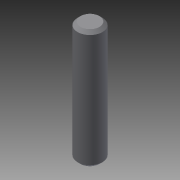
# Autodesk Inventor part: FO-020.751.194NT-00_rod-bif
Saved by Autodesk Inventor 2014 SP2 (Build 180246200, 246)
## iProperties
Created: 2020-02-04
Part Number: FO-020.751.194NT-00_rod-bif
Material: Generic
Catalog Web Link: www.cadenas.de
Description: FO1 Basic Model Rod-Bimba FLAT-1
Vendor: BIMBA
Document SubType Name: Modeling
Designer: psadmin
Manufacturer: BIMBA
Mass: 0.949795 g
Surface Area: 6.49027 cm^2
Volume: 0.949795 cm^3
Density: 1 g/cm^3
Appearance: PSOLRGB-180-180-180
Category: PARTsolutions
Company: BIMBA
Title: FO-020.751.194NT-00_rod-bif
Author: Cadenas PARTsolutions
Comments: Bimba FLAT-1
PSOL_IDENT_0: {$CADENAS_DATA\23d-libs\bimba\bimba_brand\bimba_imperial\bimba_full_line\flat_cylinders\fo1\fo1_basi
PSOL_IDENT_1: c_model_rod.prj},304 {VTYP=3D},{NB=FO-020.751.194NT-00_rod-bif},{LINA=FO-020.751.194NT-00_rod-bif},{
PSOL_IDENT_2: NN=FO1 Basic Model Rod},{DATE=22.01.2020 09:06:03},{GEOMDATE=12.12.2018 07:59:21},{VERSION=},{LINEID=
PSOL_IDENT_3: 10},{WBVAR=STROKE,ACTING,MNTR,MNTF,HR,FS,LENGTH,STPT1,STPT2,STPT3,RT,M,W,UM,MRS,FCD,RCD},{WBNUMERIC=
PSOL_IDENT_4: STROKE,LENGTH,FCD,RCD}  {NB=FO-020.751.194NT-00_rod-bif},{LINA=FO-020.751.194NT-00_rod-bif},{KT=DUMM
PSOL_IDENT_5: Y},{PN=FO-020.751.194NT-00},{PN2=FO-020.751.194NT-00},{BORE=0.56250000},{BOREPN=02},{BORE1=0.562},{S
PSOL_IDENT_6: TROKE=0.75000},{STROKEMIN=0.61},{STROKEMAX=16},{ACTING=},{ACTINGALG='','Double Acting, Single End Ro
PSOL_IDENT_7: d [FO]', 'D'  , 'Double Acting, Double End Rod [FOD]', 'R', 'Reverse Acting [FOR]', 'S'  ,'Single Ac
PSOL_IDENT_8: ting [FOS]'},{MNTR=},{MNTF=},{MNTFALG='','Standard Counterbored Mounting Holes','2F','Trunnion Mount
PSOL_IDENT_9: , Front','3F','Threaded Mounting Holes, Front','4F','Screw Clearance Holes, Front','5','Nose Mount'}
PSOL_IDENT_10: ,{HR=},{HRALG='','N/A'},{FS=},{LENGTHALG=[0.61:100/0.001]},{LENGTH=1.19400},{STPT1=},{STPT1ALG= '' ,
PSOL_IDENT_11: 'N/A' },{STPT2=},{STPT2ALG= '' , 'N/A' },{STPT3=},{STPT3ALG= '' , 'N/A' },{RT=NT},{M=},{W=},{UM=},{
PSOL_IDENT_12: MRS=},{MRSALG='','None ','Z','Metallic Rod Scraper [Z]'},{MALG='','Without Magnetic Position Sensing'
PSOL_IDENT_13: ,'M','With Magnetic Position Sensing [M]','M1','With Magnetic Position Sensing 1 [M1]','M3','With Ma
PSOL_IDENT_14: gnetic Position Sensing 3 [M3]' },{EE=},{EEALG='','Without Extra Extension','EE','With Extra Extensi
PSOL_IDENT_15: on'},{EELALG=0},{EELMAX=19.25},{EEL=0},{EELPN=},{A=1.12000000},{BA=0.56000},{BB=0.69000},{BC=0.81},{
PSOL_IDENT_16: BD=1.06},{C=0.88000000},{DD=2.00000000},{D=0.11200000},{CPIL=0.12000000},{DC=0.18800000},{DCP=0.1200
PSOL_IDENT_17: 0000},{DCD=0.85500000},{ES=0.16400000},{EC=0.16400000},{ED=0.46000000},{F=0.25000000},{H=0.21650000}
PSOL_IDENT_18: ,{J=0.34000000},{J2=0.340},{K=0.14000000},{L=0.19000000},{LDP=0.20000000},{LP=0.16000000},{LPDP=0.28
PSOL_IDENT_19: 000000},{TD=0.65700000},{TDDP=0.10000},{TD1=0.59500},{TD2=0.61000},{TDIN=0.56200},{LSF=0.31250000},{
PSOL_IDENT_20: LSFDP=0.02000000},{BC1=0.81000},{BC2=1.38000},{BC3=1.96000},{BC4=2.52000},{BD1=1.06000},{BD2=1.62000
PSOL_IDENT_21: },{BD3=2.14000},{BD4=2.70000},{MT=0.16400000},{CMT=0.16400000},{LG=0.37500000},{HF=0.14000000},{HM=0
PSOL_IDENT_22: .00000000},{HD=},{HALG=0},{HDY=0},{HDH=1.194},{LG1=0.00000000},{FCD=0},{RCD=0},{NPT=0.000},{FTL1=0.4
PSOL_IDENT_23: 60},{FTLSR=0.360},{TDD=0.554},{TDDSR=0.454},{TDDSRC=0.000},{TDDC=0.585},{NPTTDD=0.000},{FTL=0.460},{
PSOL_IDENT_24: TDDR=0.554},{TDDRC=0.585},{WD=0.236},{TL=0.135},{HRID=0.116},{HRNTP=0.000},{HRMT=0.000},{GL=0.050},{
PSOL_IDENT_25: GD=0.115},{GR=0.019},{GLC=0.066},{GDC=0.126},{GRC=0.034},{NR=1.000},{RTALG='', 'Standard', 'CFT', 'C
PSOL_IDENT_26: oarse Female Thread', 'CMT'  , 'Male Rod Thread (Coarse)','MT', 'Male Rod End (Fine)', 'NT'  , 'Non-
PSOL_IDENT_27: Threaded Rod'},{RDEEP=0},{LDEEP=0.554},{DEEP2=0.554},{RL=1.57},{BBB=0.56},{RL22=0.125},{FSADD=0},{HD
PSOL_IDENT_28: ADD=0},{MADD=0},{AC2=0},{MADD1=0.88},{HDADD1=0.130},{FSADD1=0.250},{UMALG='','Without Magnetic Posit
PSOL_IDENT_29: ion Sensing 90','U','With Magnetic Position Sensing 90 [U]','U1','With Magnetic Position Sensing 90
PSOL_IDENT_30: Position 1 [U1]','U3','With Magnetic Position Sensing 90 Position 3 [U3]' },{FSALG='','Standard Fric
PSOL_IDENT_31: tion Seals','L','Low Friction Seals', 'X', 'Ring Rod Seal'},{MNTRALG='','Standard Counterbored Mount
PSOL_IDENT_32: ing Holes','1','Pivot Mount','1N','Pivot Mount 90 Deg. from Standard','2R','Trunnion Mount, Rear','3
PSOL_IDENT_33: R','Threaded Mounting Holes, Rear','4R','Screw Clearance Holes, Rear'},{AC1=0.380},{WALG='', 'Withou
PSOL_IDENT_34: t Wiper', 'W', 'With Wiper'},{M1=0.880},{M2=0.625},{M3=0.375},{MNT4F=,'4F','Screw Clearance Holes, F
PSOL_IDENT_35: ront'},{FTLF=0.460},{FTLR=0.46}
NN: FO1 Basic Model Rod
NT: Bimba FLAT-1
NB: FO-020.751.194NT-00_rod-bif
NBSYN: $PN2._rod-bif
LINA: FO-020.751.194NT-00_rod-bif
PN: FO-020.751.194NT-00
BORE: 0
BOREPN: 02
BORE1: 0.562
STROKE: 0.75
ACTING: Double Acting, Single End Rod [FO]
MNTR: Standard Counterbored Mounting Holes
MNTF: Standard Counterbored Mounting Holes
HR: N/A
FS: Standard Friction Seals
LENGTH: 1.194
STPT1: N/A
STPT2: N/A
STPT3: N/A
RT: Non-Threaded Rod
M: Without Magnetic Position Sensing
W: Without Wiper
UM: Without Magnetic Position Sensing 90
A: 1.12
BA: 0.56
BB: 0.69
C: 0.88
DD: 2
D: 0.112
CPIL: 0.12
DC: 0.188
DCP: 0.12
DCD: 0.855
ES: 0.164
EC: 0.164
ED: 0.46
F: 0.25
H: 0.2165
J: 0.34
J2: 0.34
K: 0.14
L: 0.19
LDP: 0.2
LP: 0.16
LPDP: 0.28
TD: 0.657
TDDP: 0.1
TD1: 0.595
TD2: 0.61
TDIN: 0.562
LSF: 0.3125
LSFDP: 0.02
BC1: 0.81
BC2: 1.38
BC3: 1.96
BC4: 2.52
BD1: 1.06
BD2: 1.62
BD3: 2.14
BD4: 2.7
MT: 0.164
CMT: 0.164
LG: 0.375
HF: 0.14
HM: 0
FCD: 0
RCD: 0
NPT: 0
FTL1: 0.46
FTLSR: 0.36
TDD: 0.554
TDDSR: 0.454
TDDSRC: 0
TDDC: 0.585
NPTTDD: 0
WD: 0.236
TL: 0.135
HRID: 0.116
HRNTP: 0
HRMT: 0
GL: 0.05
GD: 0.115
GR: 0.019
GLC: 0.066
GDC: 0.126
GRC: 0.034
NR: 1
HDADD1: 0.13
FSADD1: 0.25
AC1: 0.38
M1: 0.88
M2: 0.625
M3: 0.375
SUPPLIER: BIMBA
ARTICLENO: FO-020.751.194NT-00_rod-bif
BOMINFO: FO-020.751.194NT-00_rod-bif
CREATOR: CADENAS GmbH
Autodesk Inventor part; units mm, degrees
sketch "Sketch_10" plane through (0, 0, 0) normal (0, 0, 1) x (1, 0, 0)
  line L0 (0, 0) -> (0, 30.3276)
  line L1 (0, 30.3276) -> (2.413, 30.3276)
  line L2 (2.413, 30.3276) -> (3.175, 29.5656)
  line L3 (3.175, 29.5656) -> (3.175, 0.762)
  line L4 (3.175, 0.762) -> (2.413, 0)
  line L5 (2.413, 0) -> (0, 0)
  line L6 (0, 0) -> (0, 30.3276)
  constraints: 14 end point
revolve "Revolution1" add sketch "Sketch_10" angle 360 about axis through (0, 0, 0) along (0, -1, 0)
ref_plane "b11_XY" through (0, 0, 0) normal (0, 1, 0) x (1, 0, 0)
ref_plane "b11_YZ" through (0, 0, 0) normal (1, 0, 0) x (0, 0, -1)
ref_plane "b11_ZX" through (0, 0, 0) normal (0, 0, -1) x (0, 1, 0)
ref_plane "b2_XY" through (0, 30.3276, 0) normal (0, 1, 0) x (1, 0, 0)
ref_plane "b2_YZ" through (0, 30.3276, 0) normal (1, 0, 0) x (0, 0, -1)
ref_plane "b2_ZX" through (0, 30.3276, 0) normal (0, 0, -1) x (0, 1, 0)
ref_plane "f1_XY" through (0, 30.3276, 3.175) normal (1, 0, 0) x (0, 0, -1)
ref_plane "f1_YZ" through (0, 30.3276, 3.175) normal (0, 0, -1) x (0, 1, 0)
ref_plane "f1_ZX" through (0, 30.3276, 3.175) normal (0, 1, 0) x (1, 0, 0)
ref_plane "f2_XY" through (0, 30.3276, -3.175) normal (1, 0, 0) x (0, 0, -1)
ref_plane "f2_YZ" through (0, 30.3276, -3.175) normal (0, 0, -1) x (0, 1, 0)
ref_plane "f2_ZX" through (0, 30.3276, -3.175) normal (0, 1, 0) x (1, 0, 0)
ref_plane "h1_XY" through (-2.7496, 30.3276, 0) normal (0, 1, 0) x (1, 0, 0)
ref_plane "h1_YZ" through (-2.7496, 30.3276, 0) normal (1, 0, 0) x (0, 0, -1)
ref_plane "h1_ZX" through (-2.7496, 30.3276, 0) normal (0, 0, -1) x (0, 1, 0)
ref_plane "h2_XY" through (2.7496, 30.3276, 0) normal (0, 1, 0) x (1, 0, 0)
ref_plane "h2_YZ" through (2.7496, 30.3276, 0) normal (1, 0, 0) x (0, 0, -1)
ref_plane "h2_ZX" through (2.7496, 30.3276, 0) normal (0, 0, -1) x (0, 1, 0)
ref_plane "npt1_XY" through (0, 30.3276, 0) normal (0, 1, 0) x (1, 0, 0)
ref_plane "npt1_YZ" through (0, 30.3276, 0) normal (1, 0, 0) x (0, 0, -1)
ref_plane "npt1_ZX" through (0, 30.3276, 0) normal (0, 0, -1) x (0, 1, 0)
ref_plane "npt1_1_XY" through (0, 0, 0) normal (0, 1, 0) x (1, 0, 0)
ref_plane "npt1_1_YZ" through (0, 0, 0) normal (1, 0, 0) x (0, 0, -1)
ref_plane "npt1_1_ZX" through (0, 0, 0) normal (0, 0, -1) x (0, 1, 0)
ref_plane "npt2_XY" through (0, 30.3276, 0) normal (0, 1, 0) x (1, 0, 0)
ref_plane "npt2_YZ" through (0, 30.3276, 0) normal (1, 0, 0) x (0, 0, -1)
ref_plane "npt2_ZX" through (0, 30.3276, 0) normal (0, 0, -1) x (0, 1, 0)
ref_plane "npt2_1_XY" through (0, 0, 0) normal (0, 1, 0) x (1, 0, 0)
ref_plane "npt2_1_YZ" through (0, 0, 0) normal (1, 0, 0) x (0, 0, -1)
ref_plane "npt2_1_ZX" through (0, 0, 0) normal (0, 0, -1) x (0, 1, 0)
ref_plane "rod_XY" through (0, 0, 0) normal (0, 1, 0) x (1, 0, 0)
ref_plane "rod_YZ" through (0, 0, 0) normal (1, 0, 0) x (0, 0, -1)
ref_plane "rod_ZX" through (0, 0, 0) normal (0, 0, -1) x (0, 1, 0)
ref_plane "rod_to_part_XY" through (0, 0, 0) normal (0, 1, 0) x (1, 0, 0)
ref_plane "rod_to_part_YZ" through (0, 0, 0) normal (1, 0, 0) x (0, 0, -1)
ref_plane "rod_to_part_ZX" through (0, 0, 0) normal (0, 0, -1) x (0, 1, 0)
ref_plane "th1_XY" through (0, 30.3276, 2.0828) normal (0, 1, 0) x (1, 0, 0)
ref_plane "th1_YZ" through (0, 30.3276, 2.0828) normal (1, 0, 0) x (0, 0, -1)
ref_plane "th1_ZX" through (0, 30.3276, 2.0828) normal (0, 0, -1) x (0, 1, 0)
ref_plane "th2_XY" through (0, 30.3276, -2.0828) normal (0, 1, 0) x (1, 0, 0)
ref_plane "th2_YZ" through (0, 30.3276, -2.0828) normal (1, 0, 0) x (0, 0, -1)
ref_plane "th2_ZX" through (0, 30.3276, -2.0828) normal (0, 0, -1) x (0, 1, 0)
ref_plane "to_rod_pivot_XY" through (0, 30.3276, 0) normal (0, 1, 0) x (1, 0, 0)
ref_plane "to_rod_pivot_YZ" through (0, 30.3276, 0) normal (1, 0, 0) x (0, 0, -1)
ref_plane "to_rod_pivot_ZX" through (0, 30.3276, 0) normal (0, 0, -1) x (0, 1, 0)
ref_plane "to_rod_pivot1_XY" through (0, 0, 0) normal (0, 1, 0) x (1, 0, 0)
ref_plane "to_rod_pivot1_YZ" through (0, 0, 0) normal (1, 0, 0) x (0, 0, -1)
ref_plane "to_rod_pivot1_ZX" through (0, 0, 0) normal (0, 0, -1) x (0, 1, 0)
body "Solid1"
